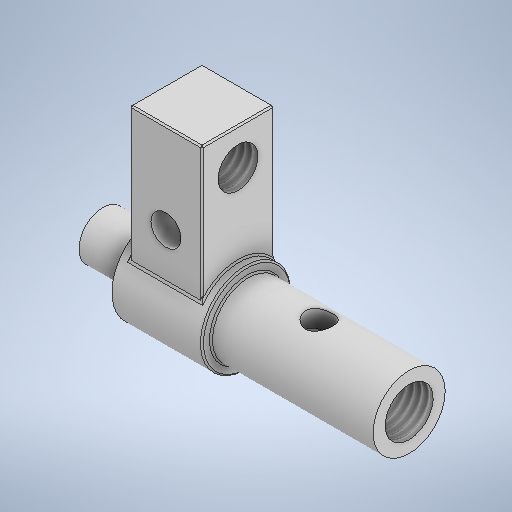
# Autodesk Inventor part: 135
Saved by Autodesk Inventor 2025.1 (Build 291241000, 241)
## iProperties
Created: 2024-08-05
Part Number: 135
Material: Generisch
Document SubType Name: Modeling
Designer: ffogue
Density: 1 g/cm^3
Appearance: Vorgabe
Author: ffogue
Autodesk Inventor part; units mm, degrees
ref_plane "YZ Plane" through (0, 0, 0) normal (1, 0, 0) x (0, 1, 0)
ref_plane "XZ Plane" through (0, 0, 0) normal (0, 1, 0) x (-1, 0, 0)
sketch "Sketch1" plane through (0, 0, 0) normal (0, 0, 1) x (1, 0, 0)
  line L0 (0, 0) -> (0, 7.5)
  line L1 (0, 7.5) -> (15, 7.5)
  line L2 (15, 7.5) -> (15, 6)
  line L3 (15, 6) -> (42, 6)
  line L4 (42, 6) -> (42, 0)
  line L5 (42, 0) -> (0, 0)
  line L6 (0, 4) -> (-9, 4)
  line L7 (-9, 4) -> (-9, 0)
  line L8 (-9, 0) -> (0, 0)
  dimension "d0" = 15
  dimension "d1" = 27
  dimension "d2" = 9
  dimension "d3" = 8
  dimension "d4" = 12
  dimension "d5" = 15
  constraints: 18 end point, 7 perpendicular, 1 horizontal, 1 point on line, 1 vertical
  measures "d0" distance of L0.end L1.end
  measures "d1" distance of L2.end L3.end
  measures "d2" distance of L6.start L6.end
  measures "d3" diameter of L6 L8
  measures "d4" diameter of L3 L5
  measures "d5" diameter of L1 L5
revolve "Revolution1" add sketch "Sketch1" angle 360 about axis through (-9, 0, 0) along (1, 0, 0)
ref_plane "Work Plane1" through (0, 0, 27) normal (0, 0, 1) x (1, 0, 0)
sketch "Sketch2" plane through (0, 0, 27) normal (0, 0, 1) x (1, 0, 0)
  line L0 (13.5, 6) -> (1.5, 6)
  line L1 (1.5, 6) -> (1.5, -6)
  line L2 (1.5, -6) -> (13.5, -6)
  line L3 (13.5, -6) -> (13.5, 6)
  line L4 (0, 7.5) -> (15, 7.5) projected
  point P0 (0, 0)
  point P1 (7.5, 6)
  point P2 (7.5, 7.5)
  point P3 (1.5, 0)
  dimension "d8" = 12
  dimension "d9" = 12
  constraints: 8 end point, 3 midpoint, 2 parallel, 1 horizontal, 1 horizontal alignment, 1 perpendicular, 1 vertical alignment
  measures "d8" distance between parallel lines of L2 L0
  measures "d9" distance between parallel lines of L1 L3
extrude "Extrusion1" add sketch "Sketch2" against normal up to surface round surface about axis through (7.5, 0, 0) along (1, 0, 0) radius 7.5 far side no
ref_plane "Work Plane2" through (0, 0, 6) normal (0, 0, 1) x (1, 0, 0)
sketch "Sketch3" plane through (0, 0, 6) normal (0, 0, 1) x (1, 0, 0)
  line L0 (42, -6) -> (42, 6) projected
  point P0 (0, 0)
  point P1 (27, 0)
  point P2 (42, 0)
  dimension "d13" = 15
  constraints: 1 horizontal alignment, 1 midpoint
  measures "d13" distance from line of L0 point (27, 0)
hole "Hole1" at (27, 0, 6) direction (0, 0, -1) diameter 4.5 end through all
sketch "Sketch4" plane through (13.5, -6, 27) normal (1, 0, 0) x (0, 0, -1)
  line L0 (0, 0) -> (0, 12) projected
  point P0 (27, 6)
  point P1 (6, 6)
  point P2 (0, 6)
  point P3 (0, 6)
  dimension "d28" = 6
  constraints: 2 midpoint, 1 horizontal alignment
  measures "d28" distance of point (0, 6) point (6, 6)
hole "Hole2" at (13.5, 0, 21) direction (-1, 0, 0) diameter 6.647 depth 8 thread size "M8x1.25" class "6H" standard "ISO Metric profile"
sketch "Sketch6" plane through (42, 0, 0) normal (1, 0, 0) x (0, 0, -1)
  circle A0 centre (0, 0) radius 6 projected
  constraints: 1 coincident
hole "Hole4" at (42, 0, 0) direction (-1, 0, 0) diameter 6.5 depth 27 counterbore diameter 8 counterbore depth 10
thread "Thread1" size "M8x1.25" class "6H" standard "ANSI Metric M Profile" length 10
sketch "Sketch8" plane through (-9, 0, 0) normal (-1, 0, 0) x (0, 0, 1)
  circle A0 centre (0, 0) radius 4 projected
  point P0 (0, 0)
  constraints: 1 coincident
hole "Hole5" at (-9, 0, 0) direction (1, 0, 0) diameter 4.5 depth 24
ref_plane "Work Plane5" through (0, 0, -7.5) normal (0, 0, 1) x (1, 0, 0)
sketch "Sketch10" plane through (0, 0, -7.5) normal (0, 0, 1) x (1, 0, 0)
  line L0 (0, -7.5) -> (0, 7.5) projected
  point P0 (0, 0)
  point P1 (7.5, 0)
  point P2 (0, 0)
  dimension "d56" = 7.5
  constraints: 1 horizontal alignment, 1 midpoint
  measures "d56" distance from line of L0 point (7.5, 0)
hole "Hole6" at (7.5, 0, -7.5) direction (0, 0, 1) diameter 2.5 depth 25
sketch "Sketch5" plane through (1.5, 6, 27) normal (0, 1, 0) x (1, 0, 0)
  line L0 (12, 0) -> (0, 0) projected
  line L1 (12, 9.3235) -> (12, 2.6765) projected
  point P0 (-1.5, 27)
  point P1 (6, 15)
  point P2 (6, 0)
  point P3 (12, 6)
  dimension "d36" = 9
  constraints: 2 midpoint, 1 vertical alignment
  measures "d36" vertical distance of point (6, 15) point (12, 6)
hole "Hole3" at (7.5, 6, 12) direction (0, -1, 0) diameter 5 end through all
chamfer "Chamfer1" distance 0.25 angle 45 10 edges at (13.5, 6, 15.75) (1.5, 6, 15.75) (7.5, 6, 4.5) (7.5, 6, 27) (1.5, 0, 27) (7.5, -6, 27) (13.5, 0, 27) (13.5, -6, 15.75) (1.5, -6, 15.75) (7.5, -6, 4.5)
chamfer "Chamfer2" distance 0.25 angle 45 2 edges at (15, -6, 0) (15, -7.5, 0)
chamfer "Chamfer3" distance 0.25 angle 45 6 edges at (1.5, 6.0742, 4.3994) (1.5, 0, 7.5) (1.5, -6.0742, 4.3994) (13.5, 6.0742, 4.3994) (13.5, 0, 7.5) (13.5, -6.0742, 4.3994)
equation "\"d9\" = d8"
body "Solid1"
